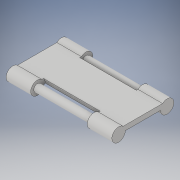
# Autodesk Inventor part: topBottomPlate
Saved by Autodesk Inventor 2019 (Build 230136000, 136)
## iProperties
Created: 2018-07-23
Part Number: topBottomPlate
Material: Generic
Document SubType Name: Modeling
Designer: Ge Shi
Density: 1 g/cm^3
Appearance: Default
Author: Ge Shi
Autodesk Inventor part; units mm, degrees
ref_plane "YZ Plane" through (0, 0, 0) normal (1, 0, 0) x (0, 1, 0)
ref_plane "XZ Plane" through (0, 0, 0) normal (0, 1, 0) x (-1, 0, 0)
ref_plane "XY Plane" through (0, 0, 0) normal (0, 0, 1) x (1, 0, 0)
sketch "Sketch1" plane through (0, 0, 0) normal (0, 1, 0) x (-1, 0, 0)
  line L0 (-21.75, 10) -> (21.75, 10)
  line L1 (21.75, 10) -> (21.75, -10)
  line L2 (21.75, -10) -> (-21.75, -10)
  line L3 (-21.75, -10) -> (-21.75, 10)
  line L4 (-21.75, 10) -> (21.75, -10) construction
  line L5 (21.75, 10) -> (-21.75, -10) construction
  point P0 (0, 0)
  dimension "d0" = 43.5
  dimension "d1" = 20
  constraints: 12 end point, 2 midpoint, 2 parallel, 1 horizontal, 1 perpendicular
  measures "d0" distance of L1.end L2.end
  measures "d1" distance of L0.end L1.end
extrude "Extrusion1" add sketch "Sketch1" along normal blind 2
ref_plane "Work Plane1" through (0, 0, 10) normal (1, 0, 0) x (0, 0, -1)
sketch "Sketch2" plane through (0, 0, 10) normal (1, 0, 0) x (0, 0, -1)
  circle A0 centre (20, 0) radius 1.5
  circle A1 centre (0, 0) radius 1.5
  circle A2 centre (0, 0) radius 2.75
  circle A3 centre (20, 0) radius 2.75
  circle A4 centre (0, 0) radius 3.25
  line L0 (20, 0) -> (0, 0) projected
  circle A5 centre (20, 0) radius 3.25
  point P0 (10, 0)
  dimension "d4" = 3
  dimension "d5" = 3
  dimension "d6" = 5.5
  dimension "d7" = 5.5
  dimension "d14" = 6.5
  dimension "d15" = 6.5
  constraints: 6 centre point, 4 coincident
  measures "d4" diameter of A0
  measures "d5" diameter of A1
  measures "d6" diameter of A2
  measures "d7" diameter of A3
  measures "d14" diameter of A4
  measures "d15" diameter of A5
extrude "Extrusion3" cut sketch "Sketch2" along normal mid plane 50 contours A0 | A1 | A2 | A3
extrude "Extrusion2" add sketch "Sketch2" along normal mid plane 43.5 contours A2 | A3
extrude "Extrusion4" cut sketch "Sketch2" along normal mid plane 23.25 contours A0 | A1 | A2 | A3 | A4 | A5
extrude "Extrusion5" add sketch "Sketch2" along normal mid plane 43.5 contours A0 | A1
equation "\"d0\" = -hingeShaftHolder + length - clearance"
equation "\"d1\" = widthOuter"
equation "\"d2\" = thick"
equation "\"d4\" = hingeShaft"
equation "\"d5\" = hingeShaft"
equation "\"d6\" = hingeShaftHolder"
equation "\"d7\" = hingeShaftHolder"
equation "\"d14\" = hingeShaftHolder + clearance"
equation "\"d15\" = hingeShaftHolder + clearance"
equation "\"d10\" = length"
equation "\"d8\" = -hingeShaftHolder + length - clearance"
equation "\"d16\" = -hingeShaftHolder + length - clearance"
equation "\"hingeShaftHolder\" = 5.5"
equation "\"length\" = 50"
equation "\"clearance\" = 1"
equation "\"widthOuter\" = 20"
equation "\"thick\" = 2"
equation "\"hingeShaft\" = 3"
body "Solid1"
